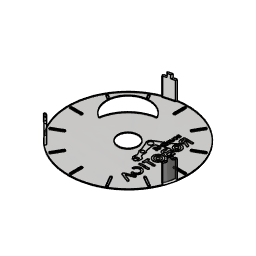
Clock v31 (Autodesk Fusion 360 archive; units mm, degrees)
design "10 quadrante"
Autodesk Fusion 360 part; units mm, degrees
(part 1 of 21)
sketch "Schizzo1" plane through (0, 0, 0) normal (0, 0, 1) x (1, 0, 0)
  circle A0 centre (0, 0) radius 60
  circle A1 centre (0, 0) radius 10
  circle A2 centre (0, 0) radius 35
  circle A3 centre (-24.0416, 24.0416) radius 21.5
  line L0 (-24.0416, 24.0416) -> (0, 0)
  line L1 (20, 0) -> (2.5, 0)
  dimension "d1" = 120
  dimension "d2" = 20
  dimension "d3" = 70
  dimension "d4" = 43
  dimension "d5" = 135
  dimension "d6" = 34
  constraint coincident A0.centre A1.centre
  constraint concentric A1 A2
  constraint coincident A3.centre L0.start
  measures "d1" diameter of A0
  measures "d2" diameter of A1
  measures "d3" diameter of A2
  measures "d4" diameter of A3
  measures "d5" angle of L0 L1
  measures "d6" distance of A3.centre A0.centre
extrude "Estrusione1" add sketch "Schizzo1" along normal blind 0.8 contours A0 | A2 A3 | A2 A3 picked at (-21.1756, -5.4075) picked at (-19.4046, 19.4046)
sketch "Schizzo2" plane through (0, 0, 0.8) normal (0, 0, 1) x (-1, 0, 0)
  arc A0 (5.3099, -34.5949) -> (34.5949, -5.3099) centre (24.0416, -24.0416) ccw
  arc A1 (5.3099, -34.5949) -> (34.5949, -5.3099) centre (0, 0) ccw
  circle A2 centre (0, 0) radius 10
  circle A3 centre (0, 0) radius 60
  circle A4 centre (0, 0) radius 60
  circle A5 centre (0, 0) radius 58
  circle A6 centre (-57.9555, 15.5291) radius 6
  circle A7 centre (42.4264, 42.4264) radius 6
  circle A8 centre (15.5291, -57.9555) radius 6
  line L0 (15.5291, -57.9555) -> (0, 0) construction
  line L1 (0, 0) -> (-57.9555, 15.5291) construction
  line L2 (0, 0) -> (42.4264, 42.4264) construction
  line L3 (-20, 0) -> (-2.5, 0)
  dimension "d9" = 116
  dimension "d10" = 12
  dimension "d11" = 12
  dimension "d12" = 12
  dimension "d15" = 120
  dimension "d16" = 120
  dimension "d17" = 120
  dimension "d18" = 75
  constraint concentric A1 A4
  constraint concentric A4 A5
  constraint coincident A3 A6.centre
  constraint coincident A4 A7.centre
  constraint coincident A4 A8.centre
  constraint coincident A8.centre L0.start
  constraint coincident A1.centre A2.centre
  constraint coincident A6.centre L1.end
  constraint coincident A7.centre L2.end
  measures "d9" diameter of A5
  measures "d10" diameter of A6
  measures "d11" diameter of A7
  measures "d12" diameter of A8
  measures "d15" angle of L0 L2
  measures "d16" angle of L0 L1
  measures "d17" diameter of A4
  measures "d18" angle of L0 L3
extrude "Estrusione2" add sketch "Schizzo2" along normal blind 18.5 contours A3 A4 A5 A7 | A3 A4 A5 A8 | A3 A4 A5 A6
sketch "Schizzo3" plane through (0, 0, 19.3) normal (0, 0, 1) x (-1, 0, 0)
  arc A0 (9.5764, -57.204) -> (9.6632, -59.2167) centre (15.5291, -57.9555) ccw
  arc A1 (9.6632, -59.2167) -> (21.2398, -56.1148) centre (0, 0) ccw
  arc A2 (21.2398, -56.1148) -> (20.3086, -54.3283) centre (15.5291, -57.9555) ccw
  arc A3 (9.5764, -57.204) -> (20.3086, -54.3283) centre (0, 0) ccw
  circle A4 centre (15.5291, -57.9555) radius 2.5
  dimension "d19" = 5
  constraint concentric A0 A4
  measures "d19" diameter of A4
extrude "Estrusione3" add sketch "Schizzo3" along normal blind 3.5 contours A1 A3 A4
pattern_circular "Serie C1" count 3 over 360 about axis through (0, 0, 1.75) along (0, 0, 1) of "Estrusione3"
sketch "Schizzo4" plane through (0, 0, 0) normal (0, 0, -1) x (1, 0, 0)
  arc A0 (-34.5949, -5.3099) -> (-5.3099, -34.5949) centre (-24.0416, -24.0416) ccw
  arc A1 (-34.5949, -5.3099) -> (-5.3099, -34.5949) centre (0, 0) ccw
  circle A2 centre (0, 0) radius 10
  circle A3 centre (0, 0) radius 60
  line L0 (-58, -0.8) -> (-46, -0.8)
  line L1 (-46, -0.8) -> (-46, 0.8)
  line L2 (-46, 0.8) -> (-58, 0.8)
  line L3 (-58, 0.8) -> (-58, -0.8)
  dimension "d24" = 0.8
  dimension "d25" = 0.8
  dimension "d26" = 58
  dimension "d27" = 12
  constraint horizontal L0
  constraint vertical L1
  constraint horizontal L2
  constraint vertical L3
  measures "d24" distance of A1.centre L0
  measures "d25" distance of A1.centre L2
  measures "d26" distance of A1.centre L3
  measures "d27" distance of L1.end L2.end
extrude "Estrusione4" cut sketch "Schizzo4" against normal blind 0.2 contours L0 L1 L2 L3
pattern_circular "Serie C2" count 12 over 360 about axis through (0, 0, 0) along (0, 0, 1) of "Estrusione4"
sketch "Schizzo5" plane through (0, 0, 0) normal (0, 0, -1) x (1, 0, 0)
  line L0 (0.8, -46) -> (0.8, -58)
  line L1 (0.8, -58) -> (-0.8, -58)
  line L2 (-0.8, -58) -> (-0.8, -46)
  line L3 (-0.8, -46) -> (0.8, -46)
  line L4 (23.6928, -39.4372) -> (29.6928, -49.8295)
  line L5 (29.6928, -49.8295) -> (28.3072, -50.6295)
  line L6 (28.3072, -50.6295) -> (22.3072, -40.2372)
  line L7 (22.3072, -40.2372) -> (23.6928, -39.4372)
  line L8 (40.2372, -22.3072) -> (50.6295, -28.3072)
  line L9 (50.6295, -28.3072) -> (49.8295, -29.6928)
  line L10 (49.8295, -29.6928) -> (39.4372, -23.6928)
  line L11 (39.4372, -23.6928) -> (40.2372, -22.3072)
  line L12 (46, 0.8) -> (58, 0.8)
  line L13 (58, 0.8) -> (58, -0.8)
  line L14 (58, -0.8) -> (46, -0.8)
  line L15 (46, -0.8) -> (46, 0.8)
  line L16 (39.4372, 23.6928) -> (49.8295, 29.6928)
  line L17 (49.8295, 29.6928) -> (50.6295, 28.3072)
  line L18 (50.6295, 28.3072) -> (40.2372, 22.3072)
  line L19 (40.2372, 22.3072) -> (39.4372, 23.6928)
  line L20 (22.3072, 40.2372) -> (28.3072, 50.6295)
  line L21 (28.3072, 50.6295) -> (29.6928, 49.8295)
  line L22 (29.6928, 49.8295) -> (23.6928, 39.4372)
  line L23 (23.6928, 39.4372) -> (22.3072, 40.2372)
  line L24 (-0.8, 46) -> (-0.8, 58)
  line L25 (-0.8, 58) -> (0.8, 58)
  line L26 (0.8, 58) -> (0.8, 46)
  line L27 (0.8, 46) -> (-0.8, 46)
  line L28 (-23.6928, 39.4372) -> (-29.6928, 49.8295)
  line L29 (-29.6928, 49.8295) -> (-28.3072, 50.6295)
  line L30 (-28.3072, 50.6295) -> (-22.3072, 40.2372)
  line L31 (-22.3072, 40.2372) -> (-23.6928, 39.4372)
  line L32 (-40.2372, 22.3072) -> (-50.6295, 28.3072)
  line L33 (-50.6295, 28.3072) -> (-49.8295, 29.6928)
  line L34 (-49.8295, 29.6928) -> (-39.4372, 23.6928)
  line L35 (-39.4372, 23.6928) -> (-40.2372, 22.3072)
  line L36 (-46, -0.8) -> (-58, -0.8)
  line L37 (-58, -0.8) -> (-58, 0.8)
  line L38 (-58, 0.8) -> (-46, 0.8)
  line L39 (-46, 0.8) -> (-46, -0.8)
  line L40 (-45.3242, -27.0917) -> (-49.8295, -29.6928)
  line L41 (-49.8295, -29.6928) -> (-50.6295, -28.3072)
  line L42 (-50.6295, -28.3072) -> (-45.502, -25.3468)
  arc A0 (-34.5949, -5.3099) -> (-45.502, -25.3468) centre (-24.0416, -24.0416) ccw
  arc A1 (-34.5949, -5.3099) -> (-5.3099, -34.5949) centre (0, 0) ccw
  arc A2 (-25.3468, -45.502) -> (-5.3099, -34.5949) centre (-24.0416, -24.0416) ccw
  line L43 (-25.3468, -45.502) -> (-28.3072, -50.6295)
  line L44 (-28.3072, -50.6295) -> (-29.6928, -49.8295)
  line L45 (-29.6928, -49.8295) -> (-27.0917, -45.3242)
  arc A3 (-45.3242, -27.0917) -> (-27.0917, -45.3242) centre (-24.0416, -24.0416) ccw
  circle A4 centre (0, 0) radius 10
  circle A5 centre (0, 0) radius 60
  circle A6 centre (0, 0) radius 35
  circle A7 centre (-24.0416, -24.0416) radius 22.5
  circle A8 centre (-24.0416, -24.0416) radius 21.5
  dimension "d32" = 45
  dimension "d37" = 43
  constraint coincident A1.centre A4.centre
  constraint concentric A3 A7
  constraint concentric A7 A8
  measures "d32" diameter of A7
  measures "d37" diameter of A8
extrude "Estrusione5" add sketch "Schizzo5" along normal up to near side of body 1 contours L40 L42 A7 A8 | L43 L45 A7 A8
sketch "Schizzo7" plane through (0, 0, 0) normal (0, 0, -1) x (1, 0, 0)
  line L0 (-46.2539, -27.6285) -> (-49.8295, -29.6928)
  line L1 (-49.8295, -29.6928) -> (-50.6295, -28.3072)
  line L2 (-50.6295, -28.3072) -> (-46.4645, -25.9026)
  arc A0 (-46.4645, -25.9026) -> (-46.2539, -27.6285) centre (-24.0416, -24.0416) ccw
  line L3 (-25.9026, -46.4645) -> (-28.3072, -50.6295)
  line L4 (-28.3072, -50.6295) -> (-29.6928, -49.8295)
  line L5 (-29.6928, -49.8295) -> (-27.6285, -46.2539)
  arc A1 (-27.6285, -46.2539) -> (-25.9026, -46.4645) centre (-24.0416, -24.0416) ccw
  line L6 (0.8, -46) -> (0.8, -58)
  line L7 (0.8, -58) -> (-0.8, -58)
  line L8 (-0.8, -58) -> (-0.8, -46)
  line L9 (-0.8, -46) -> (0.8, -46)
  line L10 (23.6928, -39.4372) -> (29.6928, -49.8295)
  line L11 (29.6928, -49.8295) -> (28.3072, -50.6295)
  line L12 (28.3072, -50.6295) -> (22.3072, -40.2372)
  line L13 (22.3072, -40.2372) -> (23.6928, -39.4372)
  line L14 (40.2372, -22.3072) -> (50.6295, -28.3072)
  line L15 (50.6295, -28.3072) -> (49.8295, -29.6928)
  line L16 (49.8295, -29.6928) -> (39.4372, -23.6928)
  line L17 (39.4372, -23.6928) -> (40.2372, -22.3072)
  line L18 (46, 0.8) -> (58, 0.8)
  line L19 (58, 0.8) -> (58, -0.8)
  line L20 (58, -0.8) -> (46, -0.8)
  line L21 (46, -0.8) -> (46, 0.8)
  line L22 (39.4372, 23.6928) -> (49.8295, 29.6928)
  line L23 (49.8295, 29.6928) -> (50.6295, 28.3072)
  line L24 (50.6295, 28.3072) -> (40.2372, 22.3072)
  line L25 (40.2372, 22.3072) -> (39.4372, 23.6928)
  line L26 (22.3072, 40.2372) -> (28.3072, 50.6295)
  line L27 (28.3072, 50.6295) -> (29.6928, 49.8295)
  line L28 (29.6928, 49.8295) -> (23.6928, 39.4372)
  line L29 (23.6928, 39.4372) -> (22.3072, 40.2372)
  line L30 (-0.8, 46) -> (-0.8, 58)
  line L31 (-0.8, 58) -> (0.8, 58)
  line L32 (0.8, 58) -> (0.8, 46)
  line L33 (0.8, 46) -> (-0.8, 46)
  line L34 (-23.6928, 39.4372) -> (-29.6928, 49.8295)
  line L35 (-29.6928, 49.8295) -> (-28.3072, 50.6295)
  line L36 (-28.3072, 50.6295) -> (-22.3072, 40.2372)
  line L37 (-22.3072, 40.2372) -> (-23.6928, 39.4372)
  line L38 (-40.2372, 22.3072) -> (-50.6295, 28.3072)
  line L39 (-50.6295, 28.3072) -> (-49.8295, 29.6928)
  line L40 (-49.8295, 29.6928) -> (-39.4372, 23.6928)
  line L41 (-39.4372, 23.6928) -> (-40.2372, 22.3072)
  line L42 (-46, -0.8) -> (-58, -0.8)
  line L43 (-58, -0.8) -> (-58, 0.8)
  line L44 (-58, 0.8) -> (-46, 0.8)
  line L45 (-46, 0.8) -> (-46, -0.8)
  circle A2 centre (0, 0) radius 12.5
  arc A3 (-34.5949, -5.3099) -> (-5.3099, -34.5949) centre (-24.0416, -24.0416) ccw
  arc A4 (-34.5949, -5.3099) -> (-5.3099, -34.5949) centre (0, 0) ccw
  circle A5 centre (0, 0) radius 60
extrude "Estrusione6" cut sketch "Schizzo7" against normal up to surface (0.8 mm away) contours L0 L1 L2 A0 | L3 L4 L5 A1 | L6 L7 L8 L9 | L10 L11 L12 L13 | L14 L15 L16 L17 | L18 L19 L20 L21 | L22 L23 L24 L25 | L26 L27 L28 L29 | L30 L31 L32 L33 | L34 L35 L36 L37 | L38 L39 L40 L41 | L42 L43 L44 L45
sketch "Schizzo8" plane through (0, 0, 0) normal (0, 0, -1) x (1, 0, 0)
  line L0 (-46.2539, -27.6285) -> (-49.8295, -29.6928)
  line L1 (-49.8295, -29.6928) -> (-50.6295, -28.3072)
  line L2 (-50.6295, -28.3072) -> (-46.4645, -25.9026)
  arc A0 (-46.4645, -25.9026) -> (-46.2539, -27.6285) centre (-24.0416, -24.0416) ccw
  line L3 (-25.9026, -46.4645) -> (-28.3072, -50.6295)
  line L4 (-28.3072, -50.6295) -> (-29.6928, -49.8295)
  line L5 (-29.6928, -49.8295) -> (-27.6285, -46.2539)
  arc A1 (-27.6285, -46.2539) -> (-25.9026, -46.4645) centre (-24.0416, -24.0416) ccw
  line L6 (0.8, -46) -> (0.8, -58)
  line L7 (0.8, -58) -> (-0.8, -58)
  line L8 (-0.8, -58) -> (-0.8, -46)
  line L9 (-0.8, -46) -> (0.8, -46)
  line L10 (23.6928, -39.4372) -> (29.6928, -49.8295)
  line L11 (29.6928, -49.8295) -> (28.3072, -50.6295)
  line L12 (28.3072, -50.6295) -> (22.3072, -40.2372)
  line L13 (22.3072, -40.2372) -> (23.6928, -39.4372)
  line L14 (40.2372, -22.3072) -> (50.6295, -28.3072)
  line L15 (50.6295, -28.3072) -> (49.8295, -29.6928)
  line L16 (49.8295, -29.6928) -> (39.4372, -23.6928)
  line L17 (39.4372, -23.6928) -> (40.2372, -22.3072)
  line L18 (46, 0.8) -> (58, 0.8)
  line L19 (58, 0.8) -> (58, -0.8)
  line L20 (58, -0.8) -> (46, -0.8)
  line L21 (46, -0.8) -> (46, 0.8)
  line L22 (39.4372, 23.6928) -> (49.8295, 29.6928)
  line L23 (49.8295, 29.6928) -> (50.6295, 28.3072)
  line L24 (50.6295, 28.3072) -> (40.2372, 22.3072)
  line L25 (40.2372, 22.3072) -> (39.4372, 23.6928)
  line L26 (22.3072, 40.2372) -> (28.3072, 50.6295)
  line L27 (28.3072, 50.6295) -> (29.6928, 49.8295)
  line L28 (29.6928, 49.8295) -> (23.6928, 39.4372)
  line L29 (23.6928, 39.4372) -> (22.3072, 40.2372)
  line L30 (-0.8, 46) -> (-0.8, 58)
  line L31 (-0.8, 58) -> (0.8, 58)
  line L32 (0.8, 58) -> (0.8, 46)
  line L33 (0.8, 46) -> (-0.8, 46)
  line L34 (-23.6928, 39.4372) -> (-29.6928, 49.8295)
  line L35 (-29.6928, 49.8295) -> (-28.3072, 50.6295)
  line L36 (-28.3072, 50.6295) -> (-22.3072, 40.2372)
  line L37 (-22.3072, 40.2372) -> (-23.6928, 39.4372)
  line L38 (-40.2372, 22.3072) -> (-50.6295, 28.3072)
  line L39 (-50.6295, 28.3072) -> (-49.8295, 29.6928)
  line L40 (-49.8295, 29.6928) -> (-39.4372, 23.6928)
  line L41 (-39.4372, 23.6928) -> (-40.2372, 22.3072)
  line L42 (-46, -0.8) -> (-58, -0.8)
  line L43 (-58, -0.8) -> (-58, 0.8)
  line L44 (-58, 0.8) -> (-46, 0.8)
  line L45 (-46, 0.8) -> (-46, -0.8)
  circle A2 centre (0, 0) radius 10
  arc A3 (-34.5949, -5.3099) -> (-5.3099, -34.5949) centre (-24.0416, -24.0416) ccw
  arc A4 (-34.5949, -5.3099) -> (-5.3099, -34.5949) centre (0, 0) ccw
  circle A5 centre (0, 0) radius 60
  line L46 (30.2119, -3.1399) -> (29.0001, -2.8965)
  line L47 (28.7382, -0.0232) -> (28.8546, -0.592)
  line L48 (34.9742, 21.3319) -> (34.76, 22.9876)
  line L49 (29.7224, -6.7727) -> (28.9525, -6.3519)
  line L50 (27.3412, -1.2376) -> (27.0925, -0.0232)
  line L51 (27.3412, 1.186) -> (28.0027, 2.1703)
  line L52 (13.876, 2.0845) -> (14.0897, 0.8905)
  line L53 (31.2376, -19.6327) -> (31.548, -19.1737)
  line L54 (16.6365, 7.7332) -> (16.4365, 7.0332)
  line L55 (33.1831, -5.8334) -> (31.9455, -5.6052)
  line L56 (18.0197, -0.4009) -> (18.5867, 0.0042)
  line L57 (31.1442, -4.6937) -> (32.056, -4.4126)
  line L58 (32.0639, -22.9837) -> (32.8741, -22.5441)
  line L59 (30.6484, 26.3002) -> (29.1456, 26.1943)
  line L60 (33.1937, -8.0241) -> (33.2916, -8.5057)
  line L61 (27.3412, -19.814) -> (27.0979, -18.6035)
  line L62 (31.9343, 29.2768) -> (30.876, 29.6816)
  line L63 (29.6325, -19.9462) -> (30.2013, -20.0574)
  line L64 (32.9847, 22.9744) -> (33.2345, 22.2904)
  line L65 (16.4864, -7.5062) -> (17.7365, -0.6668)
  line L66 (28.5715, 28.7952) -> (30.3045, 28.1311)
  line L67 (14.1114, 0.8944) -> (10.9145, -6.7953)
  line L68 (32.4052, 19.3761) -> (31.4131, 18.712)
  line L69 (33.3154, 21.5668) -> (33.0693, 20.363)
  line L70 (34.1541, -2.6866) -> (34.5933, -1.8753)
  line L71 (29.7833, 30.1049) -> (28.7065, 30.5203)
  line L72 (32.8727, 17.6125) -> (33.5826, 18.1933)
  line L73 (19.6075, 6.2514) -> (22.6879, 8.0889)
  line L74 (30.368, 33.6794) -> (28.6509, 33.0206)
  line L75 (22.3788, -18.0146) -> (21.5497, -17.8032)
  line L76 (34.7494, -7.3839) -> (34.1187, -6.4546)
  line L77 (28.3598, -22.9837) -> (29.2716, -23.2648)
  line L78 (32.8673, -3.9734) -> (33.5727, -3.392)
  line L79 (29.0636, -8.5136) -> (29.1456, -8.9105)
  line L80 (33.0667, 1.1807) -> (33.3128, -0.0284)
  line L81 (30.7807, -19.9463) -> (31.2376, -19.6327)
  line L82 (27.5423, 17.6209) -> (28.3493, 17.1827)
  line L83 (28.9525, -6.3519) -> (28.0768, -6.2276)
  line L84 (27.1719, -8.5136) -> (27.3915, -8.1882)
  line L85 (28.3493, 17.1827) -> (29.2562, 16.9012)
  line L86 (20.7205, -18.0146) -> (20.1525, -18.5827)
  line L87 (16.4365, 7.0332) -> (16.2365, 6.4332)
  line L88 (34.76, 22.9876) -> (34.1514, 24.247)
  line L89 (34.8761, 0.9221) -> (34.5933, 1.8289)
  line L90 (25.4548, 30.0017) -> (25.939, 29.8139)
  line L91 (29.1695, -19.634) -> (29.6325, -19.9462)
  line L92 (31.2332, -1.055) -> (31.548, -0.592)
  line L93 (19.0731, 9.6285) -> (17.3887, 10.1138)
  line L94 (31.548, -19.1737) -> (31.6644, -18.6035)
  line L95 (28.8546, -19.1737) -> (29.1695, -19.634)
  line L96 (19.2875, 11.2507) -> (19.8484, 11.1078)
  line L97 (33.0667, -19.814) -> (32.3999, -20.8035)
  line L98 (29.6325, 1.3236) -> (29.1695, 1.0087)
  line L99 (30.8045, -8.5057) -> (30.8998, -8.0241)
  line L100 (26.2356, 18.9229) -> (26.8306, 18.2013)
  line L101 (19.3358, 1.2234) -> (19.4477, 1.9574)
  line L102 (34.9637, 33.6609) -> (34.9637, 35.4495)
  line L103 (30.1352, 31.8009) -> (31.339, 32.2692)
  line L104 (26.8306, 18.2013) -> (27.5423, 17.6209)
  line L105 (29.9442, 24.6215) -> (30.7569, 24.5883)
  line L106 (31.4131, -21.4703) -> (30.2066, -21.7137)
  line L107 (25.4401, -0.0231) -> (25.5344, -0.9636)
  line L108 (25.939, 29.8139) -> (27.0449, 29.3853)
  line L109 (31.6644, -18.6035) -> (31.548, -18.0333)
  ellipse E0 centre (16.6365, 1.9332) end of major axis (16.6365, 3.5885) minor radius 1.6553
  line L110 (27.0952, 21.5562) -> (25.4363, 21.5562)
  line L111 (34.1187, -6.4546) -> (33.1831, -5.8334)
  line L112 (28.8546, 0.5457) -> (28.7382, -0.0232)
  line L113 (27.5422, -3.9721) -> (28.3519, -4.4126)
  line L114 (25.6427, -7.8733) -> (25.4336, -8.9105)
  line L115 (19.3631, 2.6896) -> (19.086, 3.3849)
  line L116 (32.9053, 28.9064) -> (31.9343, 29.2768)
  line L117 (27.3915, -8.1882) -> (27.7116, -7.9633)
  line L118 (28.8546, -18.0333) -> (28.7383, -18.6035)
  line L119 (33.5826, 18.1933) -> (34.1656, 18.8998)
  line L120 (27.0925, -0.0232) -> (27.3412, 1.186)
  line L121 (34.9637, 35.4495) -> (30.368, 33.6794)
  line L122 (30.2013, 16.8096) -> (31.1528, 16.8958)
  line L123 (22.6879, 8.0889) -> (22.4294, 12.6551)
  line L124 (19.0083, 3.4879) -> (19.0834, 3.5006)
  line L125 (28.6509, 33.0206) -> (27.1216, 32.4253)
  line L126 (14.0897, 0.8905) -> (14.1114, 0.8944)
  line L127 (33.2916, -8.5057) -> (33.2916, -10.9584)
  line L128 (30.2013, 1.44) -> (29.6325, 1.3236)
  line L129 (28.0064, -20.8035) -> (27.3412, -19.814)
  line L130 (25.4442, 14.7855) -> (25.4442, 13.1292)
  line L131 (28.8546, -0.592) -> (29.1695, -1.055)
  line L132 (29.1695, -1.055) -> (29.6434, -1.3691)
  line L133 (30.3045, 28.1311) -> (34.9901, 26.3346)
  line L134 (34.6012, -20.449) -> (34.8823, -19.5371)
  line L135 (29.1456, 24.4666) -> (29.9442, 24.6215)
  line L136 (25.4442, 13.1292) -> (34.969, 13.1292)
  line L137 (31.1644, -7.622) -> (31.5665, -7.3574)
  line L138 (25.8173, -1.8752) -> (26.2569, -2.6855)
  line L139 (31.4506, 24.3872) -> (32.0798, 24.0327)
  line L140 (33.2148, 25.263) -> (32.0269, 25.9694)
  line L141 (34.6039, 19.7041) -> (34.9742, 21.3319)
  line L142 (29.1695, -17.5729) -> (28.8546, -18.0333)
  line L143 (26.8378, -3.3904) -> (27.5422, -3.9721)
  line L144 (27.7593, 30.8881) -> (28.9287, 31.3352)
  line L145 (30.7278, -5.9234) -> (29.7224, -6.7727)
  line L146 (29.2716, -23.2648) -> (30.2118, -23.3585)
  line L147 (31.1528, 16.8958) -> (32.0666, 17.1747)
  line L148 (31.1521, -23.2648) -> (32.0639, -22.9837)
  line L149 (29.6434, -1.3691) -> (30.2013, -1.4784)
  line L150 (29.0001, -2.8965) -> (28.008, -2.2297)
  line L151 (27.7116, -7.9633) -> (28.1085, -7.8839)
  line L152 (19.086, 3.3849) -> (19.0083, 3.4879)
  line L153 (32.2883, -7.2813) -> (32.9291, -7.622)
  line L154 (14.2184, 3.2893) -> (13.876, 2.0845)
  line L155 (25.4363, 21.5562) -> (25.528, 20.6255)
  line L156 (16.2365, 6.4332) -> (15.055, 4.2225)
  line L157 (18.8389, 11.5854) -> (19.2875, 11.2507)
  line L158 (26.2591, -21.2454) -> (26.8464, -21.9624)
  line L159 (18.5467, 12.063) -> (18.8389, 11.5854)
  line L160 (32.8741, -22.5441) -> (33.5791, -21.9631)
  line L161 (34.969, 13.1292) -> (34.969, 14.7855)
  line L162 (31.339, 32.2692) -> (32.474, 32.7058)
  line L163 (32.9291, -7.622) -> (33.1937, -8.0241)
  line L164 (15.9181, 10.9062) -> (16.6365, 7.7332)
  line L165 (33.2916, -10.9584) -> (30.8019, -10.9584)
  line L166 (34.969, 14.7855) -> (25.4442, 14.7855)
  line L167 (31.4131, 18.712) -> (30.204, 18.4658)
  line L168 (33.0667, -17.3931) -> (33.3127, -18.6035)
  line L169 (27.1216, 32.4253) -> (25.984, 31.9835)
  line L170 (23.6953, -19.6737) -> (26.2591, -21.2454)
  line L171 (28.0768, -6.2276) -> (27.0449, -6.4498)
  line L172 (34.9796, -8.511) -> (34.7494, -7.3839)
  line L173 (28.3519, -4.4126) -> (29.2637, -4.6937)
  line L174 (34.976, -18.5969) -> (34.8823, -17.6566)
  line L175 (25.5344, 0.9173) -> (25.4401, -0.0231)
  line L176 (31.9455, -5.6052) -> (30.7278, -5.9234)
  line L177 (19.4477, 1.9574) -> (19.3631, 2.6896)
  line L178 (33.2345, 22.2904) -> (33.3154, 21.5668)
  line L179 (27.0449, 29.3853) -> (28.5715, 28.7952)
  line L180 (32.5952, 23.5574) -> (32.9847, 22.9744)
  line L181 (17.3887, 10.1138) -> (18.5094, 12.8552)
  line L182 (27.5541, -22.5456) -> (28.3598, -22.9837)
  line L183 (29.1695, 1.0087) -> (28.8546, 0.5457)
  line L184 (27.3439, 20.3577) -> (27.0952, 21.5562)
  line L185 (33.3127, -18.6035) -> (33.0667, -19.814)
  line L186 (30.8998, -8.0241) -> (31.1644, -7.622)
  line L187 (34.9901, 26.3346) -> (34.9901, 28.1126)
  line L188 (17.7365, -0.6668) -> (18.0197, -0.4009)
  line L189 (25.7979, 19.7393) -> (26.2356, 18.9229)
  line L190 (15.055, 4.2225) -> (14.2184, 3.2893)
  line L191 (28.9948, 18.712) -> (28.008, 19.3761)
  line L192 (31.548, -18.0333) -> (31.2324, -17.5721)
  line L193 (34.8823, -19.5371) -> (34.976, -18.5969)
  line L194 (25.4548, 31.7797) -> (25.4548, 30.0017)
  line L195 (25.984, 31.9835) -> (25.4548, 31.7797)
  line L196 (29.1456, 26.1943) -> (29.1456, 24.4666)
  line L197 (25.528, 20.6255) -> (25.7979, 19.7393)
  line L198 (27.0979, -18.6035) -> (27.3412, -17.393)
  line L199 (28.008, 19.3761) -> (27.3439, 20.3577)
  line L200 (26.2062, -7.024) -> (25.6427, -7.8733)
  line L201 (28.5133, -7.9633) -> (28.844, -8.1882)
  line L202 (20.7695, 9.1328) -> (19.0731, 9.6285)
  line L203 (30.876, 29.6816) -> (29.7833, 30.1049)
  line L204 (31.5665, -7.3574) -> (32.2883, -7.2813)
  line L205 (31.6644, -0.0232) -> (31.548, 0.5457)
  line L206 (28.9948, -21.4703) -> (28.0064, -20.8035)
  line L207 (22.8698, -17.6814) -> (23.4308, -18.3111)
  line L208 (32.0269, 25.9694) -> (30.6484, 26.3002)
  line L209 (18.5867, 0.0042) -> (19.037, 0.5538)
  line L210 (33.5727, -3.392) -> (34.1541, -2.6866)
  line L211 (20.1525, -18.5827) -> (19.9437, -19.4078)
  line L212 (32.4052, -2.2298) -> (31.4184, -2.8965)
  line L213 (18.933, 13.6478) -> (18.597, 13.2007)
  line L214 (28.7383, -18.6035) -> (28.8546, -19.1737)
  line L215 (20.6473, -18.8953) -> (21.0122, -18.5447)
  line L216 (26.8464, -21.9624) -> (27.5541, -22.5456)
  line L217 (34.8762, -0.9685) -> (34.969, -0.0232)
  line L218 (34.1514, 24.247) -> (33.2148, 25.263)
  line L219 (34.1607, -21.2587) -> (34.6012, -20.449)
  line L220 (32.0798, 24.0327) -> (32.5952, 23.5574)
  line L221 (20.4199, 11.1978) -> (20.8962, 11.4915)
  line L222 (28.9287, 31.3352) -> (30.1352, 31.8009)
  line L223 (32.0666, 17.1747) -> (32.8727, 17.6125)
  line L224 (27.0449, -6.4498) -> (26.2062, -7.024)
  line L225 (19.037, 0.5538) -> (19.3358, 1.2234)
  line L226 (29.2562, 16.9012) -> (30.2013, 16.8096)
  line L227 (30.8019, -10.9584) -> (30.8045, -8.5057)
  line L228 (20.8962, 11.4915) -> (21.2322, 11.9387)
  line L229 (28.7065, 30.5203) -> (27.7593, 30.8881)
  line L230 (32.3999, -20.8035) -> (31.4131, -21.4703)
  line L231 (34.9901, 28.1126) -> (32.9053, 28.9064)
  line L232 (25.8173, 1.8289) -> (25.5344, 0.9173)
  line L233 (27.0925, -8.9105) -> (27.1719, -8.5136)
  line L234 (29.2637, -4.6937) -> (30.204, -4.7875)
  line L235 (26.2569, -2.6855) -> (26.8378, -3.3904)
  line L236 (30.2013, -20.0574) -> (30.7807, -19.9463)
  line L237 (21.297, 12.0354) -> (20.7695, 9.1328)
  line L238 (32.474, 32.7058) -> (34.9637, 33.6609)
  line L239 (30.2066, -21.7137) -> (28.9948, -21.4703)
  line L240 (33.0693, 20.363) -> (32.4052, 19.3761)
  line L241 (19.8484, 11.1078) -> (20.4199, 11.1978)
  line L242 (20.8622, -25.6597) -> (20.966, -25.4937)
  line L243 (29.0001, -15.7368) -> (30.2119, -15.4933)
  line L244 (31.4131, -15.7368) -> (32.3999, -16.4035)
  line L245 (20.6528, -26.8694) -> (20.5253, -26.3936)
  line L246 (25.4442, -26.8572) -> (25.4442, -31.1355)
  line L247 (23.1556, -19.4064) -> (22.9468, -18.5826)
  line L248 (25.4336, -12.6147) -> (27.0925, -12.6147)
  line L249 (34.969, -29.4792) -> (27.0925, -29.4792)
  line L250 (33.5799, -15.2314) -> (32.8672, -14.6438)
  line L251 (25.4442, -31.1355) -> (34.969, -31.1355)
  line L252 (29.2637, -13.921) -> (28.3519, -14.2022)
  line L253 (29.053, -26.4471) -> (29.1351, -26.8439)
  line L254 (22.9329, -27.1499) -> (23.1547, -26.3411)
  line L255 (30.7807, -1.3646) -> (31.2332, -1.055)
  line L256 (33.2307, -25.1056) -> (32.519, -25.4152)
  line L257 (34.5933, -1.8753) -> (34.8762, -0.9685)
  line L258 (21.5443, -18.4141) -> (22.0737, -18.5446)
  line L259 (23.7112, -19.4092) -> (23.6953, -19.6737)
  line L260 (29.7648, -24.7431) -> (28.9975, -24.3304)
  line L261 (28.9975, -24.3304) -> (28.0341, -24.1836)
  line L262 (22.5504, -25.1966) -> (22.34, -25.3122)
  line L263 (20.1525, -20.2329) -> (20.7206, -20.8011)
  line L264 (20.718, -25.1375) -> (20.5034, -25.2077)
  line L265 (20.7198, -27.7261) -> (21.545, -27.9232)
  line L266 (22.349, -25.69) -> (22.5196, -25.9905)
  line L267 (22.9468, -18.5826) -> (22.3788, -18.0146)
  line L268 (32.3999, -16.4035) -> (33.0667, -17.3931)
  line L269 (27.0925, -29.4792) -> (27.0925, -26.9021)
  line L270 (28.0341, -24.1836) -> (27.082, -24.3912)
  line L271 (18.5094, 12.8552) -> (18.4541, 12.6371)
  line L272 (30.2119, -15.4933) -> (31.4131, -15.7368)
  line L273 (23.1547, -26.3411) -> (23.0599, -25.7756)
  line L274 (20.0783, -25.739) -> (19.9388, -26.3969)
  line L275 (27.3412, -17.393) -> (28.0087, -16.4027)
  line L276 (30.204, -4.7875) -> (31.1442, -4.6937)
  line L277 (20.6473, -19.9204) -> (20.5153, -19.4078)
  line L278 (20.9162, -25.2821) -> (20.718, -25.1375)
  line L279 (31.4184, -2.8965) -> (30.2119, -3.1399)
  line L280 (19.9834, 14.0315) -> (19.4092, 13.9415)
  line L281 (29.1456, -12.6147) -> (34.9796, -12.6147)
  line L282 (34.969, -31.1355) -> (34.969, -29.4792)
  line L283 (20.9914, 13.5526) -> (20.5469, 13.8886)
  line L284 (30.204, 18.4658) -> (28.9948, 18.712)
  line L285 (19.0834, 3.5006) -> (19.6075, 6.2514)
  line L286 (28.1085, -7.8839) -> (28.5133, -7.9633)
  line L287 (28.844, -8.1882) -> (29.0636, -8.5136)
  line L288 (30.2118, -23.3585) -> (31.1521, -23.2648)
  line L289 (25.5344, -0.9636) -> (25.8173, -1.8752)
  line L290 (33.5791, -21.9631) -> (34.1607, -21.2587)
  line L291 (34.1656, 18.8998) -> (34.6039, 19.7041)
  line L292 (28.008, -2.2297) -> (27.3412, -1.2376)
  line L293 (30.7569, 24.5883) -> (31.4506, 24.3872)
  line L294 (22.0848, -27.1894) -> (21.5542, -27.3129)
  line L295 (20.5469, 13.8886) -> (19.9834, 14.0315)
  line L296 (28.3519, -14.2022) -> (27.7593, -14.5197)
  line L297 (32.3999, 2.1703) -> (33.0667, 1.1807)
  line L298 (29.1351, -26.8439) -> (29.1351, -28.696)
  line L299 (33.0667, -1.2376) -> (32.4052, -2.2298)
  line L300 (31.2324, -17.5721) -> (30.7702, -17.2581)
  line L301 (33.3128, -0.0284) -> (33.0667, -1.2376)
  line L302 (19.4092, 13.9415) -> (18.933, 13.6478)
  line L303 (18.021, 13.8203) -> (15.9181, 10.9062)
  line L304 (21.2851, 13.0764) -> (20.9914, 13.5526)
  line L305 (21.2322, 11.9387) -> (21.375, 12.5022)
  line L306 (18.5218, 12.9042) -> (18.021, 13.8203)
  line L307 (18.4541, 12.6371) -> (18.5467, 12.063)
  line L308 (34.6012, -16.7448) -> (34.1615, -15.9402)
  line L309 (22.0737, -18.5446) -> (22.4362, -18.8952)
  line L310 (18.597, 13.2007) -> (18.5218, 12.9042)
  line L311 (22.4363, -26.8497) -> (22.0848, -27.1894)
  line L312 (29.6325, -17.2581) -> (29.1695, -17.5729)
  line L313 (22.4362, -18.8952) -> (22.5682, -19.4065)
  line L314 (31.2331, 1.0086) -> (30.7702, 1.3236)
  line L315 (30.2013, -17.139) -> (29.6325, -17.2581)
  line L316 (32.056, -14.2022) -> (31.1442, -13.921)
  line L317 (22.9469, -20.2329) -> (23.1556, -19.4064)
  line L318 (30.7702, -17.2581) -> (30.2013, -17.139)
  line L319 (30.2013, -1.4784) -> (30.7807, -1.3646)
  line L320 (21.375, 12.5022) -> (21.2851, 13.0764)
  line L321 (20.5253, -26.3936) -> (20.6046, -26.0015)
  line L322 (31.548, -0.592) -> (31.6644, -0.0232)
  line L323 (28.0087, -16.4027) -> (29.0001, -15.7368)
  line L324 (34.969, -0.0232) -> (34.8761, 0.9221)
  line L325 (22.4294, 12.6551) -> (21.297, 12.0354)
  line L326 (30.7702, 1.3236) -> (30.2013, 1.44)
  line L327 (32.056, -4.4126) -> (32.8673, -3.9734)
  line L328 (23.4308, -18.3111) -> (23.7112, -19.4092)
  line L329 (31.548, 0.5457) -> (31.2331, 1.0086)
  line L330 (30.204, -13.8273) -> (29.2637, -13.921)
  line L331 (19.9437, -19.4078) -> (20.1525, -20.2329)
  line L332 (22.34, -25.3122) -> (22.2737, -25.5153)
  line L333 (28.3002, -25.8458) -> (28.8334, -26.1269)
  line L334 (27.0925, -26.9021) -> (27.1587, -26.4841)
  line L335 (34.1529, 2.6387) -> (33.5712, 3.3431)
  line L336 (25.4336, -8.9105) -> (25.4336, -12.6147)
  line L337 (21.5497, -17.8032) -> (20.7205, -18.0146)
  line L338 (34.9796, -12.6147) -> (34.9796, -8.511)
  line L339 (18.7833, -7.563) -> (18.6995, -7.7943)
  line L340 (32.519, -25.4152) -> (31.8179, -25.7221)
  line L341 (34.8823, -17.6566) -> (34.6012, -16.7448)
  line L342 (22.0735, -20.2737) -> (21.5443, -20.4042)
  line L343 (25.4336, 5.3029) -> (27.0925, 5.3029)
  line L344 (31.1442, -13.921) -> (30.204, -13.8273)
  line L345 (20.5153, -19.4078) -> (20.6473, -18.8953)
  line L346 (20.1508, -27.1855) -> (20.7198, -27.7261)
  line L347 (21.5913, -7.4823) -> (18.9996, -7.4823)
  line L348 (22.7551, -25.276) -> (22.5504, -25.1966)
  line L349 (30.7199, -26.1957) -> (30.3601, -25.3781)
  line L350 (29.2637, 4.6448) -> (28.3519, 4.3636)
  line L351 (30.4421, -28.1272) -> (31.3919, -27.7091)
  line L352 (22.2737, -25.5153) -> (22.349, -25.69)
  line L353 (22.5196, -25.9905) -> (22.5696, -26.3382)
  line L354 (29.1456, -8.9105) -> (29.1456, -12.6147)
  line L355 (21.5418, -10.7067) -> (22.3654, -10.5009)
  line L356 (34.1615, -15.9402) -> (33.5799, -15.2314)
  line L357 (32.8672, -14.6438) -> (32.056, -14.2022)
  line L358 (21.0173, -27.1963) -> (20.6528, -26.8694)
  line L359 (27.0925, 9.0335) -> (27.0925, 11.1052)
  line L360 (31.1988, -25.9867) -> (30.7199, -26.1957)
  line L361 (22.3655, -27.7174) -> (22.9329, -27.1499)
  line L362 (21.0124, -20.2736) -> (20.6473, -19.9204)
  line L363 (31.8179, -25.7221) -> (31.1988, -25.9867)
  line L364 (28.3519, 4.3636) -> (27.5427, 3.9235)
  line L365 (27.0925, -12.6147) -> (27.0925, -8.9105)
  line L366 (32.8662, 3.9241) -> (32.056, 4.3636)
  line L367 (20.966, -25.4937) -> (20.9162, -25.2821)
  line L368 (21.0122, -18.5447) -> (21.5443, -18.4141)
  line L369 (28.8334, -26.1269) -> (29.053, -26.4471)
  line L370 (22.5696, -26.3382) -> (22.4363, -26.8497)
  line L371 (20.0381, -6.5679) -> (20.2516, -6.6452)
  line L372 (27.0925, 11.1052) -> (25.4336, 11.1052)
  line L373 (27.082, -24.3912) -> (26.2274, -24.9654)
  line L374 (26.2574, 2.6382) -> (25.8173, 1.8289)
  line L375 (19.9388, -26.3969) -> (20.1508, -27.1855)
  line L376 (29.6483, -28.4738) -> (30.4421, -28.1272)
  line L377 (31.3919, -27.7091) -> (32.3973, -27.262)
  line L378 (30.3601, -25.3781) -> (29.7648, -24.7431)
  line L379 (20.6046, -26.0015) -> (20.8622, -25.6597)
  line L380 (22.4361, -19.9206) -> (22.0735, -20.2737)
  line L381 (21.545, -27.9232) -> (22.3655, -27.7174)
  line L382 (19.9504, -6.3326) -> (20.0381, -6.5679)
  line L383 (19.4793, -6.0359) -> (19.1918, -5.9183)
  line L384 (20.5034, -25.2077) -> (20.0783, -25.739)
  line L385 (19.6046, -6.3319) -> (19.5798, -6.2817)
  line L386 (21.5497, -21.0098) -> (22.3787, -20.8011)
  line L387 (34.969, 9.0335) -> (27.0925, 9.0335)
  line L388 (26.2274, -24.9654) -> (25.6532, -25.82)
  line L389 (22.8318, -6.6451) -> (23.0461, -6.5675)
  line L390 (22.4337, -9.6175) -> (22.0678, -9.9738)
  line L391 (28.9948, 2.837) -> (30.2066, 3.0804)
  line L392 (27.3703, -26.1428) -> (27.7011, -25.9126)
  line L393 (34.969, 7.3772) -> (34.969, 9.0335)
  line L394 (21.5443, -20.4042) -> (21.0124, -20.2736)
  line L395 (22.4337, -8.6031) -> (22.568, -9.1115)
  line L396 (22.3787, -20.8011) -> (22.9469, -20.2329)
  line L397 (27.0925, 5.3029) -> (27.0925, 7.3772)
  line L398 (20.5389, -9.3665) -> (20.5147, -8.9739)
  line L399 (18.7914, -6.3169) -> (18.8997, -6.6022)
  line L400 (23.1561, -9.1116) -> (22.933, -8.2897)
  line L401 (34.9796, -26.1349) -> (34.9796, -24.3436)
  line L402 (23.0599, -25.7756) -> (22.7551, -25.276)
  line L403 (26.8385, 3.3424) -> (26.2574, 2.6382)
  line L404 (18.7833, -8.0216) -> (18.9989, -8.1057)
  line L405 (21.5542, -27.3129) -> (21.0173, -27.1963)
  line L406 (30.2066, 3.0804) -> (31.4131, 2.837)
  line L407 (22.3676, -7.7243) -> (21.5913, -7.4823)
  line L408 (22.3654, -10.5009) -> (22.933, -9.9334)
  line L409 (29.1351, -28.696) -> (29.6483, -28.4738)
  line L410 (20.0419, -24.4994) -> (20.2438, -24.5839)
  line L411 (21.7698, -21.7348) -> (21.7698, -21.709)
  line L412 (34.5933, 1.8289) -> (34.1529, 2.6387)
  line L413 (22.4606, -23.5414) -> (22.1747, -23.8482)
  line L414 (22.933, -9.9334) -> (23.1561, -9.1116)
  line L415 (30.204, 4.7385) -> (29.2637, 4.6448)
  line L416 (19.9385, -9.134) -> (20.1503, -9.9331)
  line L417 (23.0446, -6.1068) -> (22.8319, -6.0298)
  line L418 (20.7206, -20.8011) -> (21.5497, -21.0098)
  line L419 (21.8561, -21.7348) -> (21.7698, -21.7348)
  line L420 (12.1315, -12.5366) -> (18.3615, -16.4194)
  line L421 (23.1236, -6.31) -> (23.0446, -6.1068)
  line L422 (32.056, 4.3636) -> (31.1442, 4.6448)
  line L423 (19.9495, -24.2785) -> (20.0419, -24.4994)
  line L424 (22.568, -9.1115) -> (22.4337, -9.6175)
  line L425 (20.7181, -10.5009) -> (21.5418, -10.7067)
  line L426 (20.2446, -23.9658) -> (20.0412, -24.0472)
  line L427 (22.0683, -8.2497) -> (22.4337, -8.6031)
  line L428 (18.9996, -7.4823) -> (18.7833, -7.563)
  line L429 (18.6995, -7.7943) -> (18.7833, -8.0216)
  line L430 (18.9989, -8.1057) -> (20.3864, -8.1056)
  line L431 (19.5798, -6.2817) -> (19.4793, -6.0359)
  line L432 (19.1918, -5.9183) -> (18.9004, -6.0406)
  line L433 (32.3973, -27.262) -> (34.9796, -26.1349)
  line L434 (23.1231, -6.3513) -> (23.1236, -6.31)
  line L435 (25.6532, -25.82) -> (25.4442, -26.8572)
  line L436 (22.933, -8.2897) -> (22.3676, -7.7243)
  line L437 (20.1503, -9.9331) -> (20.7181, -10.5009)
  line L438 (27.7011, -25.9126) -> (28.3002, -25.8458)
  line L439 (22.5682, -19.4065) -> (22.4361, -19.9206)
  line L440 (27.1587, -26.4841) -> (27.3703, -26.1428)
  line L441 (23.0461, -6.5675) -> (23.1231, -6.3513)
  line L442 (25.4336, 11.1052) -> (25.4336, 5.3029)
  line L443 (21.0125, -8.2497) -> (21.5404, -8.1192)
  line L444 (21.5404, -8.1192) -> (22.0683, -8.2497)
  line L445 (21.7698, -21.709) -> (21.8561, -21.7348)
  line L446 (22.2468, -28.2859) -> (21.7721, -28.3994)
  line L447 (20.0382, -21.716) -> (19.9503, -21.9439)
  line L448 (27.0925, 7.3772) -> (34.969, 7.3772)
  line L449 (33.5712, 3.3431) -> (32.8662, 3.9241)
  line L450 (34.9796, -24.3436) -> (33.2307, -25.1056)
  line L451 (28.0027, 2.1703) -> (28.9948, 2.837)
  line L452 (27.5427, 3.9235) -> (26.8385, 3.3424)
  line L453 (22.1812, -12.2214) -> (16.8251, -10.1325)
  line L454 (22.0678, -9.9738) -> (21.5404, -10.1091)
  line L455 (31.4131, 2.837) -> (32.3999, 2.1703)
  line L456 (20.0391, -6.1067) -> (19.9504, -6.3326)
  line L457 (22.5585, -23.0946) -> (22.4606, -23.5414)
  line L458 (23.154, -29.5475) -> (23.0382, -28.9096)
  line L459 (31.1442, 4.6448) -> (30.204, 4.7385)
  line L460 (23.1299, -21.9439) -> (23.0459, -21.7157)
  line L461 (21.5404, -10.1091) -> (21.0098, -9.973)
  line L462 (23.0459, -21.7157) -> (22.8327, -21.6348)
  line L463 (20.2516, -6.0298) -> (20.0391, -6.1067)
  line L464 (22.9874, -23.8776) -> (23.1605, -23.1368)
  line L465 (21.6856, -24.5839) -> (22.4792, -24.3973)
  line L466 (20.7139, -9.7187) -> (20.5389, -9.3665)
  line L467 (21.9608, -29.0338) -> (22.2013, -28.8978)
  line L468 (20.4196, -28.4288) -> (20.0487, -28.899)
  line L469 (20.3864, -8.1056) -> (20.1061, -8.4296)
  line L470 (20.6447, -28.3645) -> (20.4196, -28.4288)
  line L471 (22.5695, -29.5513) -> (22.4971, -29.9833)
  line L472 (22.2444, -30.7256) -> (22.4593, -30.8472)
  line L473 (18.9004, -6.0406) -> (18.7914, -6.3169)
  line L474 (27.7593, -14.5197) -> (23.6371, -12.8105)
  line L475 (20.2516, -6.6452) -> (22.8318, -6.6451)
  line L476 (22.8319, -22.2502) -> (23.0456, -22.1729)
  line L477 (20.3262, -30.5725) -> (20.857, -30.7403)
  line L478 (18.8997, -6.6022) -> (19.192, -6.7249)
  line L479 (22.8327, -21.6348) -> (20.2449, -21.6348)
  line L480 (19.4784, -6.6067) -> (19.6046, -6.3319)
  line L481 (22.7031, -13.3814) -> (22.8288, -13.3814)
  line L482 (20.5594, -29.2071) -> (20.7795, -28.9061)
  line L483 (22.9928, -22.4403) -> (22.818, -22.2502)
  line L484 (20.8787, -28.7275) -> (20.8427, -28.5035)
  line L485 (20.0487, -28.899) -> (19.916, -29.568)
  line L486 (22.465, -22.6607) -> (22.5585, -23.0946)
  line L487 (20.1061, -8.4296) -> (19.9385, -9.134)
  line L488 (21.7721, -28.3994) -> (21.4317, -28.7665)
  line L489 (19.192, -6.7249) -> (19.4784, -6.6067)
  line L490 (23.0359, -13.2963) -> (23.1192, -13.07)
  line L491 (22.3696, -14.9779) -> (22.0705, -15.2356)
  line L492 (20.2438, -24.5839) -> (21.6856, -24.5839)
  line L493 (20.644, -8.6061) -> (21.0125, -8.2497)
  line L494 (23.1234, -16.3697) -> (23.0497, -16.1348)
  line L495 (23.0391, -30.2171) -> (23.154, -29.5475)
  line L496 (22.9332, -15.209) -> (23.1452, -14.4089)
  line L497 (23.0456, -22.1729) -> (23.1299, -21.9439)
  line L498 (23.0382, -28.9096) -> (22.7052, -28.4538)
  line L499 (23.1605, -23.1368) -> (22.9928, -22.4403)
  line L500 (20.857, -30.7403) -> (21.4573, -30.4402)
  line L501 (21.0098, -9.973) -> (20.7139, -9.7187)
  line L502 (21.4317, -28.7665) -> (21.2232, -29.4441)
  line L503 (23.0497, -16.1348) -> (22.8257, -16.0348)
  line L504 (20.2449, -21.6348) -> (20.0382, -21.716)
  line L505 (23.7112, -14.4138) -> (23.6407, -14.9745)
  line L506 (19.916, -29.568) -> (20.0158, -30.1379)
  line L507 (19.9503, -21.9439) -> (20.0385, -22.1725)
  line L508 (22.1813, -30.4892) -> (22.2444, -30.7256)
  line L509 (21.4573, -30.4402) -> (21.7736, -29.6077)
  line L510 (20.2457, -22.2502) -> (21.8856, -22.2502)
  line L511 (21.7736, -29.6077) -> (21.9608, -29.0338)
  line L512 (23.4758, -15.7844) -> (23.6848, -16.377)
  line L513 (22.2183, -22.3604) -> (22.465, -22.6607)
  line L514 (22.2705, -30.3144) -> (22.1813, -30.4892)
  line L515 (20.5147, -8.9739) -> (20.644, -8.6061)
  line L516 (23.1234, -16.4608) -> (23.1234, -16.3697)
  line L517 (23.4228, -15.496) -> (23.3197, -15.6441)
  line L518 (20.0385, -22.1725) -> (20.2457, -22.2502)
  line L519 (20.8341, -30.127) -> (20.6017, -29.9908)
  line L520 (23.4493, -17.2052) -> (22.8698, -17.6814)
  line L521 (21.8856, -22.2502) -> (22.2183, -22.3604)
  line L522 (22.8319, -6.0298) -> (20.2516, -6.0298)
  line L523 (20.0412, -24.0472) -> (19.9495, -24.2785)
  line L524 (23.6847, -16.4485) -> (23.4493, -17.2052)
  line L525 (20.7795, -28.9061) -> (20.8787, -28.7275)
  line L526 (22.1747, -23.8482) -> (21.6627, -23.9658)
  line L527 (22.8257, -16.0348) -> (22.595, -16.1077)
  line L528 (18.3615, -16.4194) -> (18.9965, -16.1362)
  line L529 (22.5133, -16.4178) -> (22.4012, -16.602)
  line L530 (22.818, -22.2502) -> (22.8319, -22.2502)
  line L531 (20.0158, -30.1379) -> (20.3262, -30.5725)
  line L532 (23.1452, -14.4089) -> (22.9499, -13.6503)
  line L533 (22.4468, -29.0322) -> (22.5695, -29.5513)
  line L534 (22.0704, -13.4989) -> (22.4392, -13.8628)
  line L535 (22.5689, -14.2318) -> (22.5447, -14.625)
  line L536 (23.6705, -13.1987) -> (23.5366, -13.5645)
  line L537 (23.6407, -14.9745) -> (23.4228, -15.496)
  line L538 (22.4012, -16.602) -> (22.0747, -16.6819)
  line L539 (22.9499, -13.6503) -> (22.7031, -13.3814)
  line L540 (22.6835, -30.7751) -> (23.0391, -30.2171)
  line L541 (20.4396, -12.5123) -> (21.4867, -12.2536)
  line L542 (20.9261, -15.1779) -> (20.6472, -14.8766)
  line L543 (20.6472, -14.8766) -> (20.5116, -14.5039)
  line L544 (22.4593, -30.8472) -> (22.6835, -30.7751)
  line L545 (22.4792, -24.3973) -> (22.9874, -23.8776)
  line L546 (22.7052, -28.4538) -> (22.2468, -28.2859)
  line L547 (22.4971, -29.9833) -> (22.2705, -30.3144)
  line L548 (23.0359, -12.8397) -> (22.828, -12.758)
  line L549 (21.0116, -13.4998) -> (21.543, -13.3685)
  line L550 (21.6627, -23.9658) -> (20.2446, -23.9658)
  line L551 (18.7678, -17.2169) -> (18.9786, -17.2946)
  line L552 (21.1081, -29.8916) -> (20.9739, -30.0821)
  line L553 (22.2013, -28.8978) -> (22.4468, -29.0322)
  line L554 (22.8288, -13.3814) -> (23.0359, -13.2963)
  line L555 (22.9909, -16.8936) -> (23.1234, -16.4608)
  line L556 (21.2232, -29.4441) -> (21.1081, -29.8916)
  line L557 (21.6812, -15.3686) -> (21.2854, -15.3455)
  line L558 (22.0964, -17.2946) -> (22.6169, -17.1928)
  line L559 (20.9739, -30.0821) -> (20.8341, -30.127)
  line L560 (20.6017, -29.9908) -> (20.4956, -29.5757)
  line L561 (20.4956, -29.5757) -> (20.5594, -29.2071)
  line L562 (22.0747, -16.6819) -> (18.9778, -16.6818)
  line L563 (18.7678, -16.7629) -> (18.6834, -16.9879)
  line L564 (23.6371, -12.8105) -> (23.6705, -13.1987)
  line L565 (19.9383, -14.3635) -> (20.1499, -15.1849)
  line L566 (20.7178, -15.7527) -> (21.5429, -15.9639)
  line L567 (19.6687, -13.2806) -> (20.4396, -12.5123)
  line L568 (23.5366, -13.5645) -> (23.7112, -14.4138)
  line L569 (22.0705, -15.2356) -> (21.6812, -15.3686)
  line L570 (22.4392, -13.8628) -> (22.5689, -14.2318)
  line L571 (23.6848, -16.377) -> (23.6847, -16.4485)
  line L572 (23.3197, -15.6441) -> (23.4758, -15.7844)
  line L573 (22.6169, -17.1928) -> (22.9909, -16.8936)
  line L574 (20.7173, -12.9775) -> (20.15, -13.5448)
  line L575 (21.4867, -12.2536) -> (22.1812, -12.2214)
  line L576 (22.5447, -14.625) -> (22.3696, -14.9779)
  line L577 (22.828, -12.758) -> (21.5312, -12.7581)
  line L578 (21.5429, -15.9639) -> (22.3646, -15.7776)
  line L579 (19.4548, -14.9368) -> (19.386, -14.3719)
  line L580 (22.5133, -16.2984) -> (22.5133, -16.4178)
  line L581 (22.595, -16.1077) -> (22.5133, -16.2984)
  line L582 (22.3646, -15.7776) -> (22.9332, -15.209)
  line L583 (19.669, -15.4642) -> (19.4548, -14.9368)
  line L584 (23.1192, -13.07) -> (23.0359, -12.8397)
  line L585 (20.8427, -28.5035) -> (20.6447, -28.3645)
  line L586 (20.5116, -14.5039) -> (20.5342, -14.1083)
  line L587 (18.9786, -17.2946) -> (22.0964, -17.2946)
  line L588 (19.4539, -13.8069) -> (19.6687, -13.2806)
  line L589 (18.9965, -16.1362) -> (20.2906, -16.1362)
  line L590 (20.5342, -14.1083) -> (20.7112, -13.7538)
  line L591 (19.386, -14.3719) -> (19.4539, -13.8069)
  line L592 (21.2854, -15.3455) -> (20.9261, -15.1779)
  line L593 (20.2906, -16.1362) -> (19.669, -15.4642)
  line L594 (18.9778, -16.6818) -> (18.7678, -16.7629)
  line L595 (20.7112, -13.7538) -> (21.0116, -13.4998)
  line L596 (21.543, -13.3685) -> (22.0704, -13.4989)
  line L597 (21.5312, -12.7581) -> (20.7173, -12.9775)
  line L598 (20.15, -13.5448) -> (19.9383, -14.3635)
  line L599 (11.312, -8.1738) -> (11.7312, -7.6194)
  line L600 (20.1499, -15.1849) -> (20.7178, -15.7527)
  line L601 (16.8251, -10.1325) -> (16.9333, -9.3147)
  line L602 (16.9333, -9.3147) -> (16.8544, -8.4658)
  line L603 (9.9491, -9.9963) -> (10.2371, -10.8252)
  line L604 (18.6834, -16.9879) -> (18.7678, -17.2169)
  line L605 (10.3743, -7.4786) -> (10.0231, -8.269)
  line L606 (16.5833, -7.6619) -> (16.4864, -7.5062)
  line L607 (13.3502, -11.6344) -> (12.6636, -11.5258)
  line L608 (12.0512, -11.2285) -> (11.55, -10.7676)
  line L609 (15.6681, -8.8496) -> (15.6985, -9.5298)
  line L610 (14.6556, -11.2493) -> (14.0384, -11.5368)
  line L611 (12.5083, -7.1155) -> (13.3876, -6.9525)
  line L612 (11.7312, -7.6194) -> (12.5083, -7.1155)
  line L613 (15.6985, -9.5298) -> (15.5262, -10.2032)
  line L614 (10.0231, -8.269) -> (9.8774, -9.1213)
  line L615 (15.1641, -10.7965) -> (14.6556, -11.2493)
  line L616 (12.6636, -11.5258) -> (12.0512, -11.2285)
  line L617 (14.2643, -7.1296) -> (15.0332, -7.6458)
  line L618 (11.0771, -8.8129) -> (11.312, -8.1738)
  line L619 (11.55, -10.7676) -> (11.1973, -10.1686)
  line L620 (11.3546, -12.1263) -> (12.1315, -12.5366)
  line L621 (10.2371, -10.8252) -> (10.7145, -11.5456)
  line L622 (16.8544, -8.4658) -> (16.5833, -7.6619)
  line L623 (11.1973, -10.1686) -> (11.0358, -9.4925)
  line L624 (13.3876, -6.9525) -> (14.2643, -7.1296)
  line L625 (14.0384, -11.5368) -> (13.3502, -11.6344)
  line L626 (15.4434, -8.2068) -> (15.6681, -8.8496)
  line L627 (11.0358, -9.4925) -> (11.0771, -8.8129)
  line L628 (9.8774, -9.1213) -> (9.9491, -9.9963)
  line L629 (15.0332, -7.6458) -> (15.4434, -8.2068)
  line L630 (10.7145, -11.5456) -> (11.3546, -12.1263)
  line L631 (15.5262, -10.2032) -> (15.1641, -10.7965)
  line L632 (10.9145, -6.7953) -> (10.3743, -7.4786)
extrude "Estrusione7" cut sketch "Schizzo8" against normal blind 0.2 contours L47 L92 L98 L112 L128 L131 L132 L149 L183 L205 L255 L314 L319 L322 L326 L329 | L48 L59 L64 L68 L69 L72 L82 L85 L88 L100 L104 L105 L110 L119 L122 L135 L139 L140 L141 L147 L155 L167 L178 L180 L184 L189 L191 L196 L197 L199 L208 L218 L220 L223 L226 L240 L284 L291 L293 | L49 L55 L76 L79 L83 L84 L111 L114 L117 L145 L151 L171 L172 L176 L200 L201 L224 L233 L248 L281 L286 L287 L336 L338 L354 L365 | L52 L54 L56 L65 L67 L73 L87 L93 L96 L101 L115 L123 L124 L126 L152 L154 L156 L157 L159 L164 L177 L181 L188 L190 L202 L209 L213 L221 L225 L228 L237 L241 L271 L280 L283 L285 L295 L302 L303 L304 L305 L306 L307 L310 L320 L325 L420 L453 L528 L541 L567 L575 L579 L583 L588 L589 L591 L593 L601 L602 L603 L605 L606 L614 L620 L621 L622 L628 L630 L632 | L53 L63 L81 L91 L94 L95 L109 L118 L142 L192 L214 L236 L300 L312 L315 L318 | L57 L70 L78 L89 L107 L113 L138 L143 L173 L175 L210 L217 L232 L234 L235 L257 L276 L289 L324 L327 L335 L350 L364 L366 L374 L403 L412 L415 L422 L449 L452 L459 | L58 L77 L134 L146 L148 L158 L160 L170 L174 L182 L193 L207 L216 L219 L250 L252 L259 L288 L290 L296 L308 L316 L328 L330 L341 L344 L356 L357 L474 L505 L512 L517 L520 L524 L536 L537 L564 L568 L571 L572 | L62 L66 L71 L74 L90 L102 L103 L108 L116 L121 L125 L133 L144 L162 L169 L179 L187 L194 L195 L203 L222 L229 L231 L238 | L75 L86 L211 L247 L263 L267 L317 L331 L337 L386 L396 L418 | L130 L136 L161 L166 | L242 L245 L254 L262 L264 L265 L266 L273 L274 L278 L294 L311 L321 L332 L346 L348 L352 L353 L358 L361 L367 L370 L375 L379 L381 L384 L402 L405 | L246 L249 L251 L253 L256 L260 L261 L269 L270 L282 L298 L333 L334 L340 L349 L351 L360 L363 L369 L373 L376 L377 L378 L388 L392 L401 L409 L433 L435 L438 L440 L450 | L339 L347 L355 L400 L404 L407 L408 L414 L416 L425 L428 L429 L430 L436 L437 L469 L487 | L343 L359 L372 L387 L393 L397 L442 L448 | L371 L382 L389 L417 L421 L434 L441 L456 L463 L475 L522 | L383 L385 L399 L431 L432 L473 L478 L480 L489 | L410 L413 L423 L426 L447 L457 L460 L462 L464 L465 L476 L479 L483 L486 L492 L497 L499 L504 L507 L510 L513 L518 L521 L523 L526 L530 L545 L550 | L446 L458 L467 L468 L470 L471 L472 L477 L482 L484 L485 L488 L495 L498 L500 L502 L506 L508 L509 L511 L514 L519 L525 L531 L533 L540 L544 L546 L547 L552 L553 L556 L559 L560 L561 L585 | L481 L490 L496 L532 L539 L548 L554 L565 L566 L574 L577 L578 L582 L584 L597 L598 L600 | L494 L503 L516 L527 L529 L538 L551 L555 L558 L562 L563 L573 L580 L581 L587 L594 L604

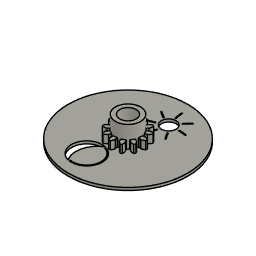
design "9 night and day"
description: Spur Gear; Module: 1.000000; Num Teeth: 12; Pressure Angle: 20.000000; Backlash: 0.00 mm
Autodesk Fusion 360 part; units mm, degrees
sketch "Schizzo1" plane through (0, 0, 0) normal (0, 0, 1) x (1, 0, 0)
  circle A0 centre (0, 0) radius 22.5
  dimension "d1" = 45
  constraint coincident A0.centre origin
  measures "d1" diameter of A0
extrude "Estrusione1" add sketch "Schizzo1" along normal blind 1 makes body 1
sketch "Schizzo1 (2)" plane through (0, 0, 0) normal (0, 0, 1) x (1, 0, 0) in component "Spur Gear (12 teeth)"
  circle A0 centre (0, 0) radius 4.7492
extrude "Estrusione1'" add sketch "Schizzo1 (2)" along normal blind 5 separate body makes body 2 in component "Spur Gear (12 teeth)"